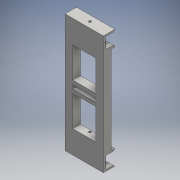
# Autodesk Inventor part: Raket_Lednings_Holder
Saved by Autodesk Inventor 2016 (Build 200138000, 138)
## iProperties
Created: 2017-08-14
Part Number: Raket_Lednings_Holder
Material: Generic
Document SubType Name: Modeling
Designer: andre
Density: 1 g/cm^3
Appearance: Default
Author: andre
Autodesk Inventor part; units mm, degrees
ref_plane "YZ Plane" through (0, 0, 0) normal (1, 0, 0) x (0, 1, 0)
ref_plane "XZ Plane" through (0, 0, 0) normal (0, 1, 0) x (-1, 0, 0)
ref_plane "XY Plane" through (0, 0, 0) normal (0, 0, 1) x (1, 0, 0)
sketch "Sketch1" plane through (0, 0, 0) normal (0, 1, 0) x (-1, 0, 0)
  line L0 (0, 0) -> (50, 0)
  line L1 (50, 0) -> (50, -155)
  line L2 (50, -155) -> (0, -155)
  line L3 (0, -155) -> (0, 0)
  dimension "d0" = 50
  dimension "d1" = 155
  constraints: 8 end point, 2 parallel, 1 horizontal, 1 perpendicular
  measures "d0" distance of L1.end L2.end
  measures "d1" distance of L0.end L1.end
extrude "Extrusion1" add sketch "Sketch1" along normal blind 10
sketch "Sketch2" plane through (0, 10, 0) normal (0, 1, 0) x (1, 0, 0)
  line L0 (0, 0) -> (0, 155) projected
  line L1 (-50, 155) -> (-50, 0) projected
  line L2 (0, 0) -> (-50, 0)
  line L3 (-50, 0) -> (-50, 20)
  line L4 (-50, 20) -> (0, 20)
  line L5 (0, 20) -> (0, 0)
  line L6 (-50, 155) -> (0, 155)
  line L7 (0, 155) -> (0, 135)
  line L8 (0, 135) -> (-50, 135)
  line L9 (-50, 135) -> (-50, 155)
  dimension "d4" = 20
  dimension "d5" = 20
  constraints: 16 end point, 4 parallel, 2 horizontal, 2 perpendicular, 2 point on line
  measures "d4" distance of L2.end L3.end
  measures "d5" distance of L6.end L7.end
extrude "Extrusion2" add sketch "Sketch2" along normal blind 5 contours L2 L1 L4 L0 | L8 L1 L6 L0
sketch "Sketch3" plane through (0, 15, 0) normal (0, 1, 0) x (1, 0, 0)
  line L0 (0, 0) -> (0, 5)
  line L1 (0, 0) -> (0, 20) projected
  line L2 (0, 5) -> (0, 15)
  line L3 (-50, 20) -> (-50, 0) projected
  line L4 (0, 13.8957) -> (-50, 13.8957)
  line L5 (-50, 13.8957) -> (-50, 5)
  line L6 (-50, 5) -> (0, 5)
  line L7 (0, 5) -> (0, 13.8957)
  line L8 (0, 155) -> (0, 0) projected
  line L9 (0, 155) -> (0, 150)
  line L10 (0, 150) -> (0, 140)
  line L11 (-50, 0) -> (-50, 155) projected
  line L12 (0, 140) -> (-50, 140)
  line L13 (-50, 155) -> (0, 155)
  line L14 (-50, 140) -> (-50, 155)
  line L15 (0, 150) -> (-50, 150)
  point P0 (-50, 195)
  dimension "d8" = 5
  dimension "d9" = 10
  dimension "d10" = 5
  dimension "d11" = 10
  constraints: 24 end point, 8 point on line, 4 horizontal, 2 parallel, 1 collinear, 1 perpendicular
  measures "d8" distance of L0.start L0.end
  measures "d9" distance of L0.end L2.end
  measures "d10" distance of L8.start L9.end
  measures "d11" distance of L9.end L10.end
extrude "Extrusion3" cut sketch "Sketch3" against normal blind 5 contours L6 L3 L4 L1 | L12 L11 L15 L8
sketch "Sketch4" plane through (0, 0, 0) normal (1, 0, 0) x (0, 0, -1)
  line L0 (13.8957, 10) -> (5, 10) projected
  line L1 (5, 10) -> (5, 0)
  line L2 (0, 0) -> (155, 0) projected
  line L3 (5, 5) -> (200, 5)
  circle A0 centre (9.4478, 5) radius 2.5
  circle A1 centre (145, 5) radius 2.5
  dimension "d44" = 5
  constraints: 4 end point, 3 point on line, 2 centre point, 1 midpoint, 1 perpendicular, 1 vertical
  measures "d44" diameter of A1
extrude "Extrusion4" cut sketch "Sketch4" against normal blind 50
sketch "Sketch5" plane through (0, 10, 0) normal (0, 1, 0) x (1, 0, 0)
  line L0 (0, 20) -> (-50, 20) projected
  line L1 (-50, 20) -> (-50, 30)
  line L2 (-50, 0) -> (-50, 155) projected
  line L3 (-50, 30) -> (-40, 30)
  line L4 (0, 135) -> (0, 125)
  line L5 (0, 125) -> (-10, 125)
  line L6 (-40, 30) -> (-10, 30)
  line L7 (-10, 30) -> (-10, 125)
  line L8 (-10, 125) -> (-40, 125)
  line L9 (-40, 125) -> (-40, 30)
  line L10 (-40, 77.5) -> (-40, 80)
  line L11 (-40, 80) -> (-10, 80)
  line L12 (-10, 80) -> (-10, 75)
  line L13 (-10, 75) -> (-40, 75)
  line L14 (-40, 75) -> (-40, 80)
  line L15 (-10, 75) -> (-10, 70)
  line L16 (-10, 80) -> (-10, 85)
  line L17 (-10, 70) -> (-40, 70)
  line L18 (-40, 70) -> (-40, 30)
  line L19 (-40, 30) -> (-10, 30)
  line L20 (-10, 30) -> (-10, 70)
  line L21 (-10, 85) -> (-40, 85)
  line L22 (-40, 85) -> (-40, 125)
  line L23 (-40, 125) -> (-10, 125)
  line L24 (-10, 125) -> (-10, 85)
  point P0 (0, 0)
  dimension "d17" = 10
  dimension "d18" = 10
  dimension "d19" = 10
  dimension "d21" = 10
  dimension "d22" = 2.5
  dimension "d23" = 5
  dimension "d24" = 5
  dimension "d25" = 5
  constraints: 46 end point, 8 parallel, 5 horizontal, 5 perpendicular, 5 point on line, 1 midpoint
  measures "d17" distance of L0.end L1.end
  measures "d18" distance of L1.end L3.end
  measures "d19" distance of L4.start L4.end
  measures "d21" distance of L4.end L5.end
  measures "d22" distance of L10.start L10.end
  measures "d23" distance of L11.end L12.end
  measures "d24" distance of L12.end L15.end
  measures "d25" distance of L11.end L16.end
extrude "Extrusion5" cut sketch "Sketch5" against normal blind 10 contours L9 L17 L7 L6 | L9 L11 L7 L13 | L21 L9 L8 L7
chamfer "Chamfer1" distance 7 angle 45 4 edges at (0, 10, -9.4478) (0, 10, -145) (-50, 10, -145) (-50, 10, -9.4478)
chamfer "Chamfer2" distance 5 angle 45 4 edges at (-25, 15, -13.8957) (-25, 15, -140) (-25, 15, -5) (-25, 15, -150)
chamfer "Chamfer3" distance 3 angle 45 8 edges at (0, 6.5, -140) (0, 6.5, -5) (-50, 6.5, -5) (-50, 6.5, -140) (-50, 6.5, -13.8957) (0, 6.5, -13.8957) (-50, 6.5, -150) (0, 6.5, -150)
sketch "Sketch6" plane through (-50, 0, 0) normal (0, 0, 1) x (1, 0, 0)
  line L0 (45.5, 7.5) -> (4.5, 7.5) projected
  circle A0 centre (25, 7.5) radius 1.5
  point P0 (50, 0)
  dimension "d37" = 3
  constraints: 1 centre point, 1 midpoint
  measures "d37" diameter of A0
extrude "Extrusion6" cut sketch "Sketch6" against normal blind 40
sketch "Sketch7" plane through (0, 0, -155) normal (0, 0, -1) x (-1, 0, 0)
  circle A0 centre (25, 7.5) radius 1.5 projected
  circle A1 centre (25, 7.5) radius 1.5
  point P0 (0, 0)
  constraints: 1 centre point, 1 coincident
extrude "Extrusion7" cut sketch "Sketch7" against normal blind 30
body "Solid1"
